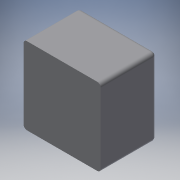
# Autodesk Inventor part: baseFoot
Saved by Autodesk Inventor 2019 (Build 230136000, 136)
## iProperties
Created: 2019-05-07
Part Number: baseFoot
Material: Generic
Document SubType Name: Modeling
Designer: Alex Jones
Density: 1 g/cm^3
Appearance: Default
Author: Alex Jones
Autodesk Inventor part; units mm, degrees
ref_plane "YZ Plane" through (0, 0, 0) normal (1, 0, 0) x (0, 1, 0)
ref_plane "XZ Plane" through (0, 0, 0) normal (0, 1, 0) x (-1, 0, 0)
ref_plane "XY Plane" through (0, 0, 0) normal (0, 0, 1) x (1, 0, 0)
sketch "Sketch1" plane through (0, 0, 0) normal (0, 0, 1) x (1, 0, 0)
  arc A0 (-10, -8.75) -> (-8.75, -10) centre (-8.75, -8.75) ccw projected
  line L0 (-8.75, -10) -> (-3.6, -10) projected
  line L1 (-3.6, -10) -> (-3.1, -9.5) projected
  line L2 (-3.1, -9.5) -> (-3.1, -8.4) projected
  line L3 (-3.1, -8.4) -> (-5.5, -8.4) projected
  line L4 (-5.5, -8.4) -> (-5.5, -6.466) projected
  line L5 (-5.5, -6.466) -> (-3.134, -4.1) projected
  line L6 (-3.134, -4.1) -> (3.134, -4.1) projected
  line L7 (3.134, -4.1) -> (5.5, -6.466) projected
  line L8 (5.5, -6.466) -> (5.5, -8.4) projected
  line L9 (5.5, -8.4) -> (3.1, -8.4) projected
  line L10 (3.1, -8.4) -> (3.1, -9.5) projected
  line L11 (3.1, -9.5) -> (3.6, -10) projected
  line L12 (3.6, -10) -> (8.75, -10) projected
  arc A1 (8.75, -10) -> (10, -8.75) centre (8.75, -8.75) ccw projected
  line L13 (10, -8.75) -> (10, -3.6) projected
  line L14 (10, -3.6) -> (9.5, -3.1) projected
  line L15 (9.5, -3.1) -> (8.4, -3.1) projected
  line L16 (8.4, -3.1) -> (8.4, -5.5) projected
  line L17 (8.4, -5.5) -> (6.466, -5.5) projected
  line L18 (6.466, -5.5) -> (4.1, -3.134) projected
  line L19 (4.1, -3.134) -> (4.1, 3.134) projected
  line L20 (4.1, 3.134) -> (6.466, 5.5) projected
  line L21 (6.466, 5.5) -> (8.4, 5.5) projected
  line L22 (8.4, 5.5) -> (8.4, 3.1) projected
  line L23 (8.4, 3.1) -> (9.5, 3.1) projected
  line L24 (9.5, 3.1) -> (10, 3.6) projected
  line L25 (10, 3.6) -> (10, 8.75) projected
  arc A2 (10, 8.75) -> (8.75, 10) centre (8.75, 8.75) ccw projected
  line L26 (8.75, 10) -> (3.6, 10) projected
  line L27 (3.6, 10) -> (3.1, 9.5) projected
  line L28 (3.1, 9.5) -> (3.1, 8.4) projected
  line L29 (3.1, 8.4) -> (5.5, 8.4) projected
  line L30 (5.5, 8.4) -> (5.5, 6.466) projected
  line L31 (5.5, 6.466) -> (3.134, 4.1) projected
  line L32 (3.134, 4.1) -> (-3.134, 4.1) projected
  line L33 (-3.134, 4.1) -> (-5.5, 6.466) projected
  line L34 (-5.5, 6.466) -> (-5.5, 8.4) projected
  line L35 (-5.5, 8.4) -> (-3.1, 8.4) projected
  line L36 (-3.1, 8.4) -> (-3.1, 9.5) projected
  line L37 (-3.1, 9.5) -> (-3.6, 10) projected
  line L38 (-3.6, 10) -> (-8.75, 10) projected
  arc A3 (-8.75, 10) -> (-10, 8.75) centre (-8.75, 8.75) ccw projected
  line L39 (-10, 8.75) -> (-10, 3.6) projected
  line L40 (-10, 3.6) -> (-9.5, 3.1) projected
  line L41 (-9.5, 3.1) -> (-8.4, 3.1) projected
  line L42 (-8.4, 3.1) -> (-8.4, 5.5) projected
  line L43 (-8.4, 5.5) -> (-6.466, 5.5) projected
  line L44 (-6.466, 5.5) -> (-4.1, 3.134) projected
  line L45 (-4.1, 3.134) -> (-4.1, -3.134) projected
  line L46 (-4.1, -3.134) -> (-6.466, -5.5) projected
  line L47 (-6.466, -5.5) -> (-8.4, -5.5) projected
  line L48 (-8.4, -5.5) -> (-8.4, -3.1) projected
  line L49 (-8.4, -3.1) -> (-9.5, -3.1) projected
  line L50 (-9.5, -3.1) -> (-10, -3.6) projected
  line L51 (-10, -3.6) -> (-10, -8.75) projected
  circle A4 centre (0, 0) radius 2.5 projected
  line L52 (-16.6875, 16.6875) -> (-16.6875, -16.6875)
  line L53 (-16.6875, -16.6875) -> (16.6875, -16.6875)
  line L54 (16.6875, -16.6875) -> (16.6875, 16.6875)
  line L55 (16.6875, 16.6875) -> (-16.6875, 16.6875)
  line L56 (-8.75, 10.1306) -> (-3.5459, 10.1306)
  line L57 (3.5459, 10.1306) -> (8.75, 10.1306)
  arc A5 (10.1306, 8.75) -> (8.75, 10.1306) centre (8.75, 8.75) ccw
  line L58 (10.1306, 8.75) -> (10.1306, 3.5459)
  line L59 (10.1306, -3.5459) -> (10.1306, -8.75)
  arc A6 (8.75, -10.1306) -> (10.1306, -8.75) centre (8.75, -8.75) ccw
  line L60 (8.75, -10.1306) -> (3.5459, -10.1306)
  line L61 (-3.5459, -10.1306) -> (-8.75, -10.1306)
  arc A7 (-10.1306, -8.75) -> (-8.75, -10.1306) centre (-8.75, -8.75) ccw
  line L62 (-10.1306, -8.75) -> (-10.1306, -3.5459)
  line L63 (-10.1306, 3.5459) -> (-10.1306, 8.75)
  arc A8 (-8.75, 10.1306) -> (-10.1306, 8.75) centre (-8.75, 8.75) ccw
  line L64 (-10.1306, 3.5459) -> (-10.1306, -3.5459)
  line L65 (10.1306, 3.5459) -> (10.1306, -3.5459)
  line L66 (3.5459, 10.1306) -> (-3.5459, 10.1306)
  line L67 (-3.5459, -10.1306) -> (3.5459, -10.1306)
  line L68 (10.1306, 10.1306) -> (-10.1306, 10.1306)
  line L69 (-10.1306, 10.1306) -> (-10.1306, -10.1306)
  line L70 (-10.1306, -10.1306) -> (10.1306, -10.1306)
  line L71 (10.1306, -10.1306) -> (10.1306, 10.1306)
  line L72 (10.1306, 10.1306) -> (-10.1306, -10.1306) construction
  line L73 (-10.1306, 10.1306) -> (10.1306, -10.1306) construction
  constraints: 44 end point, 8 point on circle, 5 parallel, 4 centre point, 2 horizontal, 2 midpoint, 2 perpendicular, 7 other
extrude "Extrusion1" add sketch "Sketch1" against normal blind 12.7 contours L55 L54 L53 L52
sketch "Sketch2" plane through (0, 0, 0) normal (0, 0, 1) x (1, 0, 0)
  line L0 (-16.6875, -16.6875) -> (-16.6875, 16.6875) projected
  line L1 (16.6875, -16.6875) -> (-16.6875, -16.6875)
  line L2 (-16.6875, -16.6875) -> (-16.6875, 16.6875)
  line L3 (-16.6875, 16.6875) -> (16.6875, 16.6875)
  line L4 (16.6875, 16.6875) -> (16.6875, -16.6875)
  line L5 (16.6875, -16.6875) -> (-16.6875, 16.6875) construction
  line L6 (-16.6875, -16.6875) -> (16.6875, 16.6875) construction
  point P0 (0, 0)
  constraints: 12 end point, 2 midpoint, 2 parallel, 1 horizontal, 1 perpendicular
extrude "Extrusion2" add sketch "Sketch2" along normal blind 6.35
fillet "Fillet1" radius 1.1906 8 edges at (16.6875, -16.6875, -3.175) (16.6875, 0, -12.7) (0, -16.6875, -12.7) (-16.6875, 0, -12.7) (-16.6875, -16.6875, -3.175) (0, 16.6875, -12.7) (-16.6875, 16.6875, -3.175) (16.6875, 16.6875, -3.175)
body "Solid1"
